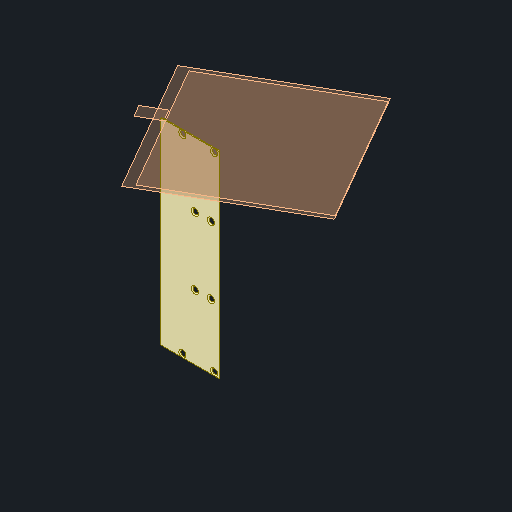
# Autodesk Inventor part: frobt
Saved by Autodesk Inventor 2023 (Build 270158000, 158)
## iProperties
Created: 2024-05-08
Part Number: frobt
Material: Nylon 6/6
Document SubType Name: Modeling
Designer: szymo
Density: 1.13 g/cm^3
Appearance: Nylon 6
Mass: 8.86148 g
Surface Area: 188.511 cm^2
Volume: 7.84202 cm^3
Author: szymo
Autodesk Inventor part; units mm, degrees
ref_plane "YZ Plane" through (0, 0, 0) normal (1, 0, 0) x (0, 1, 0)
ref_plane "Work Plane1" through (14.6553, 0, -25.7817) normal (0, 1, 0) x (-0.8660254, 0, 0.5)
ref_plane "Work Plane2" through (-53.25, -178, -67.8971) normal (0, -1, 0) x (0.8660254, 0, -0.5)
ref_plane "Work Plane3" through (14.6553, 0, -25.7817) normal (0, 1, 0) x (-0.8660254, 0, 0.5)
ref_plane "Work Plane4" through (-55.7811, 0, -1.2811) normal (0, 1, 0) x (0.5, 0, 0.8660254)
sketch "Sketch4" plane through (-55.7811, 0, -1.2811) normal (0, 1, 0) x (0.5, 0, 0.8660254)
  line L0 (3.5, 3.5) -> (-1, 3.5) projected
  line L1 (-1, 3.5) -> (-1, -0.5) projected
  line L2 (-1, -0.5) -> (-4.5, -0.5) projected
  line L3 (-4.5, -0.5) -> (-4.5, -14.5) projected
  line L4 (-4.5, -14.5) -> (4.5, -0.5) projected
  line L5 (4.5, -0.5) -> (3.5, -0.5) projected
  line L6 (3.5, -0.5) -> (3.5, 3.5) projected
  line L7 (3.5, 3.5) -> (29, 47.6673) projected
  line L8 (29, 47.6673) -> (3.5, 3.5)
  line L9 (3.5, 1.7679) -> (30, 47.6673)
  line L10 (30, 47.6673) -> (29, 47.6673)
  point P0 (29, 47.6673)
  dimension "d10" = 1
  constraints: 6 end point, 2 point on line, 1 horizontal, 1 parallel
  measures "d10" distance of L9.end L10.end
ref_plane "Work Plane5" through (-46.3218, -178, -67.8971) normal (0, -1, 0) x (0.8660254, 0, -0.5)
extrude "Extrusion2" add sketch "Sketch4" against normal up to surface (178 mm away) contours L7 L10 L9 L6
sketch "Sketch5" plane through (-52.5, 0, 0.866) normal (0, 0, 1) x (1, 0, 0)
  circle A0 centre (30.6045, -58.5) radius 2.3 projected
  circle A1 centre (45.2015, -58.5) radius 2.3 projected
  circle A2 centre (30.6045, -119.5) radius 2.3 projected
  circle A3 centre (45.2015, -119.5) radius 2.3 projected
  circle A4 centre (48, -3) radius 2 projected
  circle A5 centre (19.3979, -3) radius 2 projected
  circle A6 centre (48, -175) radius 2 projected
  circle A7 centre (19.3979, -175) radius 2 projected
  point P0 (52.5, 0)
  constraints: 8 coincident
hole "Hole2" at (-7.2985, -58.5, 0.866) at (-21.8955, -58.5, 0.866) at (-7.2985, -119.5, 0.866) at (-21.8955, -119.5, 0.866) at (-4.5, -3, 0.866) at (-33.1021, -3, 0.866) at (-4.5, -175, 0.866) at (-33.1021, -175, 0.866) direction (0, 0, -1) diameter 3.6 end through all countersink diameter 6.5 countersink angle 90 clearance for "Countersunk Flat Head Screw ISO 2009/7046" size "M3" standard "ISO"
body "Solid2"
